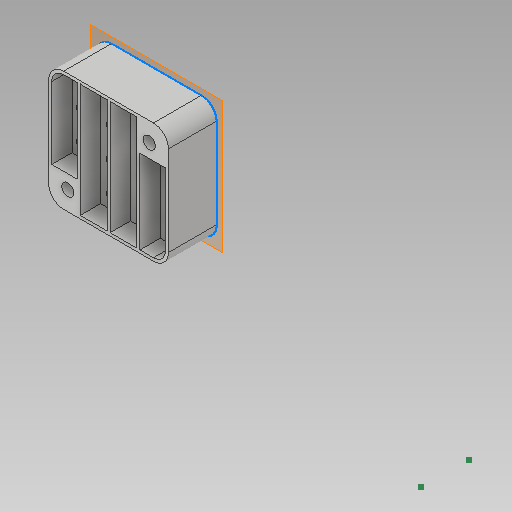
# Autodesk Inventor part: caster_wheel_1_inner
Saved by Autodesk Inventor 2019.3 (Build 233278000, 278)
## iProperties
Created: 2019-03-27
Part Number: caster_wheel_1_inner
Material: Generic
Document SubType Name: Modeling
Designer: Varga Daniel
Density: 1 g/cm^3
Appearance: Default
Author: Varga Daniel
Autodesk Inventor part; units mm, degrees
ref_plane "YZ Plane" through (0, 0, 0) normal (1, 0, 0) x (0, 1, 0)
ref_plane "XZ Plane" through (0, 0, 0) normal (0, 1, 0) x (-1, 0, 0)
ref_plane "Work Plane1" through (-90.2539, 56.452, 0) normal (0, 0, 1) x (1, 0, 0)
sketch "Sketch1" plane through (-90.2539, 56.452, 0) normal (0, 0, 1) x (1, 0, 0)
  arc A0 (0.6966, -35.7262) -> (5.6966, -30.7262) centre (0.6966, -30.7262) ccw
  line L0 (5.6966, -30.7262) -> (5.6966, -0.7262)
  arc A1 (5.6966, -0.7262) -> (0.6966, 4.2738) centre (0.6966, -0.7262) ccw
  line L1 (0.6966, 4.2738) -> (-29.3034, 4.2738)
  arc A2 (-29.3034, 4.2738) -> (-34.3034, -0.7262) centre (-29.3034, -0.7262) ccw
  line L2 (-34.3034, -0.7262) -> (-34.3034, -30.7262)
  arc A3 (-34.3034, -30.7262) -> (-29.3034, -35.7262) centre (-29.3034, -30.7262) ccw
  line L3 (-29.3034, -35.7262) -> (0.6966, -35.7262)
  line L4 (4.6966, -0.7262) -> (4.6966, -30.7262)
  arc A4 (0.6966, -34.7262) -> (4.6966, -30.7262) centre (0.6966, -30.7262) ccw
  line L5 (0.6966, -34.7262) -> (-3.8034, -34.7262)
  line L6 (-3.8034, -34.7262) -> (-3.8034, 3.2738)
  line L7 (-3.8034, 3.2738) -> (0.6966, 3.2738)
  arc A5 (4.6966, -0.7262) -> (0.6966, 3.2738) centre (0.6966, -0.7262) ccw
  line L8 (-4.8034, -34.7262) -> (-13.8034, -34.7262)
  line L9 (-13.8034, -34.7262) -> (-13.8034, 3.2738)
  line L10 (-13.8034, 3.2738) -> (-4.8034, 3.2738)
  line L11 (-4.8034, 3.2738) -> (-4.8034, -34.7262)
  line L12 (-14.8034, -34.7262) -> (-23.8034, -34.7262)
  line L13 (-23.8034, -34.7262) -> (-23.8034, 3.2738)
  line L14 (-23.8034, 3.2738) -> (-14.8034, 3.2738)
  line L15 (-14.8034, 3.2738) -> (-14.8034, -34.7262)
  line L16 (-33.3034, -30.7262) -> (-33.3034, -0.7262)
  arc A6 (-29.3034, 3.2738) -> (-33.3034, -0.7262) centre (-29.3034, -0.7262) ccw
  line L17 (-29.3034, 3.2738) -> (-24.8034, 3.2738)
  line L18 (-24.8034, 3.2738) -> (-24.8034, -34.7262)
  line L19 (-24.8034, -34.7262) -> (-29.3034, -34.7262)
  arc A7 (-33.3034, -30.7262) -> (-29.3034, -34.7262) centre (-29.3034, -30.7262) ccw
  line L20 (-28.8034, -7.2621) -> (-28.8034, -4.1903)
  arc A8 (-28.8034, -4.1903) -> (-25.8393, -1.2262) centre (-29.3034, -0.7262) ccw
  line L21 (-25.8393, -1.2262) -> (-24.8034, -1.2262)
  line L22 (-24.8034, -0.2262) -> (-24.8034, -1.2262)
  line L23 (-24.8034, -0.2262) -> (-25.8393, -0.2262)
  arc A9 (-25.8393, -0.2262) -> (-28.8034, 2.7379) centre (-29.3034, -0.7262) ccw
  line L24 (-28.8034, 2.7379) -> (-28.8034, 3.2738)
  line L25 (-29.3034, 3.2738) -> (-28.8034, 3.2738)
  arc A10 (-29.3034, 3.2738) -> (-29.8034, 3.2424) centre (-29.3034, -0.7262) ccw
  line L26 (-29.8034, 3.2424) -> (-29.8034, 2.7379)
  arc A11 (-29.8034, 2.7379) -> (-32.7675, -0.2262) centre (-29.3034, -0.7262) ccw
  line L27 (-32.7675, -0.2262) -> (-33.272, -0.2262)
  arc A12 (-33.272, -0.2262) -> (-33.3034, -0.7262) centre (-29.3034, -0.7262) ccw
  line L28 (-33.3034, -1.2262) -> (-33.3034, -0.7262)
  line L29 (-33.3034, -1.2262) -> (-32.7675, -1.2262)
  arc A13 (-32.7675, -1.2262) -> (-29.8034, -4.1903) centre (-29.3034, -0.7262) ccw
  line L30 (-29.8034, -4.1903) -> (-29.8034, -7.2621)
  arc A14 (-29.8034, -7.2621) -> (-32.7675, -10.2262) centre (-29.3034, -10.7262) ccw
  line L31 (-32.7675, -10.2262) -> (-33.3034, -10.2262)
  line L32 (-33.3034, -11.2262) -> (-33.3034, -10.2262)
  line L33 (-33.3034, -11.2262) -> (-32.7675, -11.2262)
  arc A15 (-32.7675, -11.2262) -> (-29.8034, -14.1903) centre (-29.3034, -10.7262) ccw
  line L34 (-29.8034, -14.1903) -> (-29.8034, -17.2621)
  arc A16 (-29.8034, -17.2621) -> (-32.7675, -20.2262) centre (-29.3034, -20.7262) ccw
  line L35 (-32.7675, -20.2262) -> (-33.3034, -20.2262)
  line L36 (-33.3034, -21.2262) -> (-33.3034, -20.2262)
  line L37 (-33.3034, -21.2262) -> (-32.7675, -21.2262)
  arc A17 (-32.7675, -21.2262) -> (-29.8034, -24.1903) centre (-29.3034, -20.7262) ccw
  line L38 (-29.8034, -24.1903) -> (-29.8034, -27.2621)
  arc A18 (-29.8034, -27.2621) -> (-32.7675, -30.2262) centre (-29.3034, -30.7262) ccw
  line L39 (-32.7675, -30.2262) -> (-33.3034, -30.2262)
  line L40 (-33.3034, -30.7262) -> (-33.3034, -30.2262)
  arc A19 (-33.3034, -30.7262) -> (-33.272, -31.2262) centre (-29.3034, -30.7262) ccw
  line L41 (-33.272, -31.2262) -> (-32.7675, -31.2262)
  arc A20 (-32.7675, -31.2262) -> (-29.8034, -34.1903) centre (-29.3034, -30.7262) ccw
  line L42 (-29.8034, -34.1903) -> (-29.8034, -34.6949)
  arc A21 (-29.8034, -34.6949) -> (-29.3034, -34.7262) centre (-29.3034, -30.7262) ccw
  line L43 (-28.8034, -34.7262) -> (-29.3034, -34.7262)
  line L44 (-28.8034, -34.7262) -> (-28.8034, -34.1903)
  arc A22 (-28.8034, -34.1903) -> (-25.8393, -31.2262) centre (-29.3034, -30.7262) ccw
  line L45 (-25.8393, -31.2262) -> (-24.8034, -31.2262)
  line L46 (-24.8034, -30.2262) -> (-24.8034, -31.2262)
  line L47 (-24.8034, -30.2262) -> (-25.8393, -30.2262)
  arc A23 (-25.8393, -30.2262) -> (-28.8034, -27.2621) centre (-29.3034, -30.7262) ccw
  line L48 (-28.8034, -27.2621) -> (-28.8034, -24.1903)
  arc A24 (-28.8034, -24.1903) -> (-25.8393, -21.2262) centre (-29.3034, -20.7262) ccw
  line L49 (-25.8393, -21.2262) -> (-24.8034, -21.2262)
  line L50 (-24.8034, -20.2262) -> (-24.8034, -21.2262)
  line L51 (-24.8034, -20.2262) -> (-25.8393, -20.2262)
  arc A25 (-25.8393, -20.2262) -> (-28.8034, -17.2621) centre (-29.3034, -20.7262) ccw
  line L52 (-28.8034, -17.2621) -> (-28.8034, -14.1903)
  arc A26 (-28.8034, -14.1903) -> (-25.8393, -11.2262) centre (-29.3034, -10.7262) ccw
  line L53 (-25.8393, -11.2262) -> (-24.8034, -11.2262)
  line L54 (-24.8034, -10.2262) -> (-24.8034, -11.2262)
  line L55 (-24.8034, -10.2262) -> (-25.8393, -10.2262)
  arc A27 (-25.8393, -10.2262) -> (-28.8034, -7.2621) centre (-29.3034, -10.7262) ccw
  circle A28 centre (-29.3034, -10.7262) radius 2.5
  circle A29 centre (-29.3034, -20.7262) radius 2.5
  circle A30 centre (-29.3034, -30.7262) radius 2.5
  circle A31 centre (-29.3034, -0.7262) radius 2.5
  line L56 (-22.7675, -0.2262) -> (-23.8034, -0.2262)
  line L57 (-23.8034, -1.2262) -> (-23.8034, -0.2262)
  line L58 (-23.8034, -1.2262) -> (-22.7675, -1.2262)
  arc A32 (-22.7675, -1.2262) -> (-19.8034, -4.1903) centre (-19.3034, -0.7262) ccw
  line L59 (-19.8034, -4.1903) -> (-19.8034, -7.2621)
  arc A33 (-19.8034, -7.2621) -> (-22.7675, -10.2262) centre (-19.3034, -10.7262) ccw
  line L60 (-22.7675, -10.2262) -> (-23.8034, -10.2262)
  line L61 (-23.8034, -11.2262) -> (-23.8034, -10.2262)
  line L62 (-23.8034, -11.2262) -> (-22.7675, -11.2262)
  arc A34 (-22.7675, -11.2262) -> (-19.8034, -14.1903) centre (-19.3034, -10.7262) ccw
  line L63 (-19.8034, -14.1903) -> (-19.8034, -17.2621)
  arc A35 (-19.8034, -17.2621) -> (-22.7675, -20.2262) centre (-19.3034, -20.7262) ccw
  line L64 (-22.7675, -20.2262) -> (-23.8034, -20.2262)
  line L65 (-23.8034, -21.2262) -> (-23.8034, -20.2262)
  line L66 (-23.8034, -21.2262) -> (-22.7675, -21.2262)
  arc A36 (-22.7675, -21.2262) -> (-19.8034, -24.1903) centre (-19.3034, -20.7262) ccw
  line L67 (-19.8034, -24.1903) -> (-19.8034, -27.2621)
  arc A37 (-19.8034, -27.2621) -> (-22.7675, -30.2262) centre (-19.3034, -30.7262) ccw
  line L68 (-22.7675, -30.2262) -> (-23.8034, -30.2262)
  line L69 (-23.8034, -31.2262) -> (-23.8034, -30.2262)
  line L70 (-23.8034, -31.2262) -> (-22.7675, -31.2262)
  arc A38 (-22.7675, -31.2262) -> (-19.8034, -34.1903) centre (-19.3034, -30.7262) ccw
  line L71 (-19.8034, -34.1903) -> (-19.8034, -34.7262)
  line L72 (-18.8034, -34.7262) -> (-19.8034, -34.7262)
  line L73 (-18.8034, -34.7262) -> (-18.8034, -34.1903)
  arc A39 (-18.8034, -34.1903) -> (-15.8393, -31.2262) centre (-19.3034, -30.7262) ccw
  line L74 (-15.8393, -31.2262) -> (-14.8034, -31.2262)
  line L75 (-14.8034, -30.2262) -> (-14.8034, -31.2262)
  line L76 (-14.8034, -30.2262) -> (-15.8393, -30.2262)
  arc A40 (-15.8393, -30.2262) -> (-18.8034, -27.2621) centre (-19.3034, -30.7262) ccw
  line L77 (-18.8034, -27.2621) -> (-18.8034, -24.1903)
  arc A41 (-18.8034, -24.1903) -> (-15.8393, -21.2262) centre (-19.3034, -20.7262) ccw
  line L78 (-15.8393, -21.2262) -> (-14.8034, -21.2262)
  line L79 (-14.8034, -20.2262) -> (-14.8034, -21.2262)
  line L80 (-14.8034, -20.2262) -> (-15.8393, -20.2262)
  arc A42 (-15.8393, -20.2262) -> (-18.8034, -17.2621) centre (-19.3034, -20.7262) ccw
  line L81 (-18.8034, -17.2621) -> (-18.8034, -14.1903)
  arc A43 (-18.8034, -14.1903) -> (-15.8393, -11.2262) centre (-19.3034, -10.7262) ccw
  line L82 (-15.8393, -11.2262) -> (-14.8034, -11.2262)
  line L83 (-14.8034, -10.2262) -> (-14.8034, -11.2262)
  line L84 (-14.8034, -10.2262) -> (-15.8393, -10.2262)
  arc A44 (-15.8393, -10.2262) -> (-18.8034, -7.2621) centre (-19.3034, -10.7262) ccw
  line L85 (-18.8034, -7.2621) -> (-18.8034, -4.1903)
  arc A45 (-18.8034, -4.1903) -> (-15.8393, -1.2262) centre (-19.3034, -0.7262) ccw
  line L86 (-15.8393, -1.2262) -> (-14.8034, -1.2262)
  line L87 (-14.8034, -0.2262) -> (-14.8034, -1.2262)
  line L88 (-14.8034, -0.2262) -> (-15.8393, -0.2262)
  arc A46 (-15.8393, -0.2262) -> (-18.8034, 2.7379) centre (-19.3034, -0.7262) ccw
  line L89 (-18.8034, 2.7379) -> (-18.8034, 3.2738)
  line L90 (-19.8034, 3.2738) -> (-18.8034, 3.2738)
  line L91 (-19.8034, 3.2738) -> (-19.8034, 2.7379)
  arc A47 (-19.8034, 2.7379) -> (-22.7675, -0.2262) centre (-19.3034, -0.7262) ccw
  circle A48 centre (-19.3034, -10.7262) radius 2.5
  circle A49 centre (-19.3034, -20.7262) radius 2.5
  circle A50 centre (-19.3034, -30.7262) radius 2.5
  circle A51 centre (-19.3034, -0.7262) radius 2.5
  line L92 (-12.7675, -0.2262) -> (-13.8034, -0.2262)
  line L93 (-13.8034, -1.2262) -> (-13.8034, -0.2262)
  line L94 (-13.8034, -1.2262) -> (-12.7675, -1.2262)
  arc A52 (-12.7675, -1.2262) -> (-9.8034, -4.1903) centre (-9.3034, -0.7262) ccw
  line L95 (-9.8034, -4.1903) -> (-9.8034, -7.2621)
  arc A53 (-9.8034, -7.2621) -> (-12.7675, -10.2262) centre (-9.3034, -10.7262) ccw
  line L96 (-12.7675, -10.2262) -> (-13.8034, -10.2262)
  line L97 (-13.8034, -11.2262) -> (-13.8034, -10.2262)
  line L98 (-13.8034, -11.2262) -> (-12.7675, -11.2262)
  arc A54 (-12.7675, -11.2262) -> (-9.8034, -14.1903) centre (-9.3034, -10.7262) ccw
  line L99 (-9.8034, -14.1903) -> (-9.8034, -17.2621)
  arc A55 (-9.8034, -17.2621) -> (-12.7675, -20.2262) centre (-9.3034, -20.7262) ccw
  line L100 (-12.7675, -20.2262) -> (-13.8034, -20.2262)
  line L101 (-13.8034, -21.2262) -> (-13.8034, -20.2262)
  line L102 (-13.8034, -21.2262) -> (-12.7675, -21.2262)
  arc A56 (-12.7675, -21.2262) -> (-9.8034, -24.1903) centre (-9.3034, -20.7262) ccw
  line L103 (-9.8034, -24.1903) -> (-9.8034, -27.2621)
  arc A57 (-9.8034, -27.2621) -> (-12.7675, -30.2262) centre (-9.3034, -30.7262) ccw
  line L104 (-12.7675, -30.2262) -> (-13.8034, -30.2262)
  line L105 (-13.8034, -31.2262) -> (-13.8034, -30.2262)
  line L106 (-13.8034, -31.2262) -> (-12.7675, -31.2262)
  arc A58 (-12.7675, -31.2262) -> (-9.8034, -34.1903) centre (-9.3034, -30.7262) ccw
  line L107 (-9.8034, -34.1903) -> (-9.8034, -34.7262)
  line L108 (-8.8034, -34.7262) -> (-9.8034, -34.7262)
  line L109 (-8.8034, -34.7262) -> (-8.8034, -34.1903)
  arc A59 (-8.8034, -34.1903) -> (-5.8393, -31.2262) centre (-9.3034, -30.7262) ccw
  line L110 (-5.8393, -31.2262) -> (-4.8034, -31.2262)
  line L111 (-4.8034, -30.2262) -> (-4.8034, -31.2262)
  line L112 (-4.8034, -30.2262) -> (-5.8393, -30.2262)
  arc A60 (-5.8393, -30.2262) -> (-8.8034, -27.2621) centre (-9.3034, -30.7262) ccw
  line L113 (-8.8034, -27.2621) -> (-8.8034, -24.1903)
  arc A61 (-8.8034, -24.1903) -> (-5.8393, -21.2262) centre (-9.3034, -20.7262) ccw
  line L114 (-5.8393, -21.2262) -> (-4.8034, -21.2262)
  line L115 (-4.8034, -20.2262) -> (-4.8034, -21.2262)
  line L116 (-4.8034, -20.2262) -> (-5.8393, -20.2262)
  arc A62 (-5.8393, -20.2262) -> (-8.8034, -17.2621) centre (-9.3034, -20.7262) ccw
  line L117 (-8.8034, -17.2621) -> (-8.8034, -14.1903)
  arc A63 (-8.8034, -14.1903) -> (-5.8393, -11.2262) centre (-9.3034, -10.7262) ccw
  line L118 (-5.8393, -11.2262) -> (-4.8034, -11.2262)
  line L119 (-4.8034, -10.2262) -> (-4.8034, -11.2262)
  line L120 (-4.8034, -10.2262) -> (-5.8393, -10.2262)
  arc A64 (-5.8393, -10.2262) -> (-8.8034, -7.2621) centre (-9.3034, -10.7262) ccw
  line L121 (-8.8034, -7.2621) -> (-8.8034, -4.1903)
  arc A65 (-8.8034, -4.1903) -> (-5.8393, -1.2262) centre (-9.3034, -0.7262) ccw
  line L122 (-5.8393, -1.2262) -> (-4.8034, -1.2262)
  line L123 (-4.8034, -0.2262) -> (-4.8034, -1.2262)
  line L124 (-4.8034, -0.2262) -> (-5.8393, -0.2262)
  arc A66 (-5.8393, -0.2262) -> (-8.8034, 2.7379) centre (-9.3034, -0.7262) ccw
  line L125 (-8.8034, 2.7379) -> (-8.8034, 3.2738)
  line L126 (-9.8034, 3.2738) -> (-8.8034, 3.2738)
  line L127 (-9.8034, 3.2738) -> (-9.8034, 2.7379)
  arc A67 (-9.8034, 2.7379) -> (-12.7675, -0.2262) centre (-9.3034, -0.7262) ccw
  circle A68 centre (-9.3034, -10.7262) radius 2.5
  circle A69 centre (-9.3034, -20.7262) radius 2.5
  circle A70 centre (-9.3034, -30.7262) radius 2.5
  circle A71 centre (-9.3034, -0.7262) radius 2.5
  line L128 (0.1966, -4.1903) -> (0.1966, -7.2621)
  arc A72 (0.1966, -7.2621) -> (-2.7675, -10.2262) centre (0.6966, -10.7262) ccw
  line L129 (-2.7675, -10.2262) -> (-3.8034, -10.2262)
  line L130 (-3.8034, -11.2262) -> (-3.8034, -10.2262)
  line L131 (-3.8034, -11.2262) -> (-2.7675, -11.2262)
  arc A73 (-2.7675, -11.2262) -> (0.1966, -14.1903) centre (0.6966, -10.7262) ccw
  line L132 (0.1966, -14.1903) -> (0.1966, -17.2621)
  arc A74 (0.1966, -17.2621) -> (-2.7675, -20.2262) centre (0.6966, -20.7262) ccw
  line L133 (-2.7675, -20.2262) -> (-3.8034, -20.2262)
  line L134 (-3.8034, -21.2262) -> (-3.8034, -20.2262)
  line L135 (-3.8034, -21.2262) -> (-2.7675, -21.2262)
  arc A75 (-2.7675, -21.2262) -> (0.1966, -24.1903) centre (0.6966, -20.7262) ccw
  line L136 (0.1966, -24.1903) -> (0.1966, -27.2621)
  arc A76 (0.1966, -27.2621) -> (-2.7675, -30.2262) centre (0.6966, -30.7262) ccw
  line L137 (-2.7675, -30.2262) -> (-3.8034, -30.2262)
  line L138 (-3.8034, -31.2262) -> (-3.8034, -30.2262)
  line L139 (-3.8034, -31.2262) -> (-2.7675, -31.2262)
  arc A77 (-2.7675, -31.2262) -> (0.1966, -34.1903) centre (0.6966, -30.7262) ccw
  line L140 (0.1966, -34.1903) -> (0.1966, -34.7262)
  line L141 (0.6966, -34.7262) -> (0.1966, -34.7262)
  arc A78 (0.6966, -34.7262) -> (1.1966, -34.6949) centre (0.6966, -30.7262) ccw
  line L142 (1.1966, -34.6949) -> (1.1966, -34.1903)
  arc A79 (1.1966, -34.1903) -> (4.1607, -31.2262) centre (0.6966, -30.7262) ccw
  line L143 (4.1607, -31.2262) -> (4.6652, -31.2262)
  arc A80 (4.6652, -31.2262) -> (4.6966, -30.7262) centre (0.6966, -30.7262) ccw
  line L144 (4.6966, -30.2262) -> (4.6966, -30.7262)
  line L145 (4.6966, -30.2262) -> (4.1607, -30.2262)
  arc A81 (4.1607, -30.2262) -> (1.1966, -27.2621) centre (0.6966, -30.7262) ccw
  line L146 (1.1966, -27.2621) -> (1.1966, -24.1903)
  arc A82 (1.1966, -24.1903) -> (4.1607, -21.2262) centre (0.6966, -20.7262) ccw
  line L147 (4.1607, -21.2262) -> (4.6966, -21.2262)
  line L148 (4.6966, -20.2262) -> (4.6966, -21.2262)
  line L149 (4.6966, -20.2262) -> (4.1607, -20.2262)
  arc A83 (4.1607, -20.2262) -> (1.1966, -17.2621) centre (0.6966, -20.7262) ccw
  line L150 (1.1966, -17.2621) -> (1.1966, -14.1903)
  arc A84 (1.1966, -14.1903) -> (4.1607, -11.2262) centre (0.6966, -10.7262) ccw
  line L151 (4.1607, -11.2262) -> (4.6966, -11.2262)
  line L152 (4.6966, -10.2262) -> (4.6966, -11.2262)
  line L153 (4.6966, -10.2262) -> (4.1607, -10.2262)
  arc A85 (4.1607, -10.2262) -> (1.1966, -7.2621) centre (0.6966, -10.7262) ccw
  line L154 (1.1966, -7.2621) -> (1.1966, -4.1903)
  arc A86 (1.1966, -4.1903) -> (4.1607, -1.2262) centre (0.6966, -0.7262) ccw
  line L155 (4.1607, -1.2262) -> (4.6966, -1.2262)
  line L156 (4.6966, -0.7262) -> (4.6966, -1.2262)
  arc A87 (4.6966, -0.7262) -> (4.6652, -0.2262) centre (0.6966, -0.7262) ccw
  line L157 (4.6652, -0.2262) -> (4.1607, -0.2262)
  arc A88 (4.1607, -0.2262) -> (1.1966, 2.7379) centre (0.6966, -0.7262) ccw
  line L158 (1.1966, 2.7379) -> (1.1966, 3.2424)
  arc A89 (1.1966, 3.2424) -> (0.6966, 3.2738) centre (0.6966, -0.7262) ccw
  line L159 (0.1966, 3.2738) -> (0.6966, 3.2738)
  line L160 (0.1966, 3.2738) -> (0.1966, 2.7379)
  arc A90 (0.1966, 2.7379) -> (-2.7675, -0.2262) centre (0.6966, -0.7262) ccw
  line L161 (-2.7675, -0.2262) -> (-3.8034, -0.2262)
  line L162 (-3.8034, -1.2262) -> (-3.8034, -0.2262)
  line L163 (-3.8034, -1.2262) -> (-2.7675, -1.2262)
  arc A91 (-2.7675, -1.2262) -> (0.1966, -4.1903) centre (0.6966, -0.7262) ccw
  circle A92 centre (0.6966, -10.7262) radius 2.5
  circle A93 centre (0.6966, -20.7262) radius 2.5
  circle A94 centre (0.6966, -30.7262) radius 2.5
  circle A95 centre (0.6966, -0.7262) radius 2.5
  point P0 (90.2539, -56.452)
  constraints: 316 end point, 160 point on circle, 96 centre point, 18 other
extrude "Extrusion2" add sketch "Sketch1" along normal blind 16 contours L4 L155 A86 L154 A85 L153 L151 A84 L150 A83 L149 L147 A82 L146 A81 L145 A4 L143 A79 L142 L5 L140 A77 L139 L6 L137 A76 L136 A75 L135 L133 A74 L132 A73 L131 L129 A72 L128 A91 L163 L161 A90 L160 L7 A5 L158 A88 L157 | L4 L153 A85 L154 A86 L155 | L157 A88 L158 A5 | L4 L149 A83 L150 A84 L151 | L160 A90 L161 L6 L7 | L4 L145 A81 L146 A82 L147 | L163 A91 L128 A72 L129 L6 | A4 L142 A79 L143 | L131 A73 L132 A74 L133 L6 | L5 L6 L139 A77 L140 | L135 A75 L136 A76 L137 L6 | L8 L109 A59 L110 L11 | L8 L107 A58 L106 L9 L104 A57 L103 A56 L102 L100 A55 L99 A54 L98 L96 A53 L95 A52 L94 L92 A67 L127 L10 L125 A66 L124 L11 L122 A65 L121 A64 L120 L118 A63 L117 A62 L116 L114 A61 L113 A60 L112 L110 A59 L109 | L8 L9 L106 A58 L107 | L112 A60 L113 A61 L114 L11 | L116 A62 L117 A63 L118 L11 | L9 L102 A56 L103 A57 L104 | L120 A64 L121 A65 L122 L11 | L9 L98 A54 L99 A55 L100 | L124 A66 L125 L10 L11 | L9 L94 A52 L95 A53 L96 | L9 L10 L127 A67 L92 | L12 L73 A39 L74 L15 | L12 L71 A38 L70 L13 L68 A37 L67 A36 L66 L64 A35 L63 A34 L62 L60 A33 L59 A32 L58 L56 A47 L91 L14 L89 A46 L88 L15 L86 A45 L85 A44 L84 L82 A43 L81 A42 L80 L78 A41 L77 A40 L76 L74 A39 L73 | L12 L13 L70 A38 L71 | L76 A40 L77 A41 L78 L15 | L80 A42 L81 A43 L82 L15 | L13 L66 A36 L67 A37 L68 | L84 A44 L85 A45 L86 L15 | L13 L62 A34 L63 A35 L64 | L88 A46 L89 L14 L15 | L13 L58 A32 L59 A33 L60 | L13 L14 L91 A47 L56 | L16 L39 A18 L38 A17 L37 L35 A16 L34 A15 L33 L31 A14 L30 A13 L29 A6 L27 A11 L26 L17 L24 A9 L23 L18 L21 A8 L20 A27 L55 L53 A26 L52 A25 L51 L49 A24 L48 A23 L47 L45 A22 L44 L19 A7 L42 A20 L41 | L16 L37 A17 L38 A18 L39 | L41 A20 L42 A7 | L16 L33 A15 L34 A16 L35 | L44 A22 L45 L18 L19 | L16 L29 A13 L30 A14 L31 | L47 A23 L48 A24 L49 L18 | A6 L26 A11 L27 | L51 A25 L52 A26 L53 L18 | L17 L18 L23 A9 L24 | L55 A27 L20 A8 L21 L18 | A28 | A29 | A30 | A31 | A48 | A49 | A50 | A51 | A68 | A69 | A70 | A71 | A92 | A93 | A94 | A95
extrude "Extrusion3" add sketch "Sketch1" along normal blind 16 contours L3 A3 L2 A2 L1 A1 L0 A0
extrude "Extrusion4" cut sketch "Sketch1" along normal blind 0.8 contours L4 L155 A86 L154 A85 L153 L151 A84 L150 A83 L149 L147 A82 L146 A81 L145 A4 L143 A79 L142 L5 L140 A77 L139 L6 L137 A76 L136 A75 L135 L133 A74 L132 A73 L131 L129 A72 L128 A91 L163 L161 A90 L160 L7 A5 L158 A88 L157 | L4 L153 A85 L154 A86 L155 | L157 A88 L158 A5 | L4 L149 A83 L150 A84 L151 | L160 A90 L161 L6 L7 | L4 L145 A81 L146 A82 L147 | L163 A91 L128 A72 L129 L6 | A4 L142 A79 L143 | L131 A73 L132 A74 L133 L6 | L5 L6 L139 A77 L140 | L135 A75 L136 A76 L137 L6 | L8 L109 A59 L110 L11 | L8 L107 A58 L106 L9 L104 A57 L103 A56 L102 L100 A55 L99 A54 L98 L96 A53 L95 A52 L94 L92 A67 L127 L10 L125 A66 L124 L11 L122 A65 L121 A64 L120 L118 A63 L117 A62 L116 L114 A61 L113 A60 L112 L110 A59 L109 | L8 L9 L106 A58 L107 | L112 A60 L113 A61 L114 L11 | L116 A62 L117 A63 L118 L11 | L9 L102 A56 L103 A57 L104 | L120 A64 L121 A65 L122 L11 | L9 L98 A54 L99 A55 L100 | L124 A66 L125 L10 L11 | L9 L94 A52 L95 A53 L96 | L9 L10 L127 A67 L92 | L12 L73 A39 L74 L15 | L12 L71 A38 L70 L13 L68 A37 L67 A36 L66 L64 A35 L63 A34 L62 L60 A33 L59 A32 L58 L56 A47 L91 L14 L89 A46 L88 L15 L86 A45 L85 A44 L84 L82 A43 L81 A42 L80 L78 A41 L77 A40 L76 L74 A39 L73 | L12 L13 L70 A38 L71 | L76 A40 L77 A41 L78 L15 | L80 A42 L81 A43 L82 L15 | L13 L66 A36 L67 A37 L68 | L84 A44 L85 A45 L86 L15 | L13 L62 A34 L63 A35 L64 | L88 A46 L89 L14 L15 | L13 L58 A32 L59 A33 L60 | L13 L14 L91 A47 L56 | L16 L39 A18 L38 A17 L37 L35 A16 L34 A15 L33 L31 A14 L30 A13 L29 A6 L27 A11 L26 L17 L24 A9 L23 L18 L21 A8 L20 A27 L55 L53 A26 L52 A25 L51 L49 A24 L48 A23 L47 L45 A22 L44 L19 A7 L42 A20 L41 | L16 L37 A17 L38 A18 L39 | L41 A20 L42 A7 | L16 L33 A15 L34 A16 L35 | L44 A22 L45 L18 L19 | L16 L29 A13 L30 A14 L31 | L47 A23 L48 A24 L49 L18 | A6 L26 A11 L27 | L51 A25 L52 A26 L53 L18 | L17 L18 L23 A9 L24 | L55 A27 L20 A8 L21 L18 | A28 | A29 | A30 | A31 | A48 | A49 | A50 | A51 | A68 | A69 | A70 | A71 | A92 | A93 | A94 | A95
extrude "Extrusion5" cut sketch "Sketch1" along normal blind 9.2 contours A28 | A29 | A31 | A48 | A49 | A50 | A51 | A68 | A69 | A70 | A71 | A92 | A93 | A94
sketch "Sketch2" plane through (-90.2539, 56.452, 16) normal (0, 0, 1) x (1, 0, 0)
  point P0 (90.2539, -56.452)
sketch "Sketch3" plane through (-90.2539, 56.452, 16) normal (0, 0, 1) x (1, 0, 0)
  arc A0 (-29.3034, 4.2738) -> (-34.3034, -0.7262) centre (-29.3034, -0.7262) ccw
  line L0 (-29.3034, 4.2738) -> (0.6966, 4.2738)
  arc A1 (5.6966, -0.7262) -> (0.6966, 4.2738) centre (0.6966, -0.7262) ccw
  line L1 (5.6966, -0.7262) -> (5.6966, -30.7262)
  arc A2 (0.6966, -35.7262) -> (5.6966, -30.7262) centre (0.6966, -30.7262) ccw
  line L2 (0.6966, -35.7262) -> (-29.3034, -35.7262)
  arc A3 (-34.3034, -30.7262) -> (-29.3034, -35.7262) centre (-29.3034, -30.7262) ccw
  line L3 (-34.3034, -30.7262) -> (-34.3034, -0.7262)
  line L4 (4.6966, -30.7262) -> (4.6966, -0.7262)
  arc A4 (4.6966, -0.7262) -> (0.6966, 3.2738) centre (0.6966, -0.7262) ccw
  line L5 (0.6966, 3.2738) -> (-3.8034, 3.2738)
  line L6 (-3.8034, 3.2738) -> (-3.8034, -34.7262)
  line L7 (-3.8034, -34.7262) -> (0.6966, -34.7262)
  arc A5 (0.6966, -34.7262) -> (4.6966, -30.7262) centre (0.6966, -30.7262) ccw
  line L8 (-13.8034, -34.7262) -> (-4.8034, -34.7262)
  line L9 (-4.8034, -34.7262) -> (-4.8034, 3.2738)
  line L10 (-4.8034, 3.2738) -> (-13.8034, 3.2738)
  line L11 (-13.8034, 3.2738) -> (-13.8034, -34.7262)
  line L12 (-23.8034, -34.7262) -> (-14.8034, -34.7262)
  line L13 (-14.8034, -34.7262) -> (-14.8034, 3.2738)
  line L14 (-14.8034, 3.2738) -> (-23.8034, 3.2738)
  line L15 (-23.8034, 3.2738) -> (-23.8034, -34.7262)
  line L16 (-33.3034, -0.7262) -> (-33.3034, -30.7262)
  arc A6 (-33.3034, -30.7262) -> (-29.3034, -34.7262) centre (-29.3034, -30.7262) ccw
  line L17 (-29.3034, -34.7262) -> (-24.8034, -34.7262)
  line L18 (-24.8034, -34.7262) -> (-24.8034, 3.2738)
  line L19 (-24.8034, 3.2738) -> (-29.3034, 3.2738)
  arc A7 (-29.3034, 3.2738) -> (-33.3034, -0.7262) centre (-29.3034, -0.7262) ccw
  line L20 (-28.8034, -4.1903) -> (-28.8034, -7.2621)
  arc A8 (-25.8393, -10.2262) -> (-28.8034, -7.2621) centre (-29.3034, -10.7262) ccw
  line L21 (-25.8393, -10.2262) -> (-24.8034, -10.2262)
  line L22 (-24.8034, -11.2262) -> (-24.8034, -10.2262)
  line L23 (-24.8034, -11.2262) -> (-25.8393, -11.2262)
  arc A9 (-28.8034, -14.1903) -> (-25.8393, -11.2262) centre (-29.3034, -10.7262) ccw
  line L24 (-28.8034, -14.1903) -> (-28.8034, -17.2621)
  arc A10 (-25.8393, -20.2262) -> (-28.8034, -17.2621) centre (-29.3034, -20.7262) ccw
  line L25 (-25.8393, -20.2262) -> (-24.8034, -20.2262)
  line L26 (-24.8034, -21.2262) -> (-24.8034, -20.2262)
  line L27 (-24.8034, -21.2262) -> (-25.8393, -21.2262)
  arc A11 (-28.8034, -24.1903) -> (-25.8393, -21.2262) centre (-29.3034, -20.7262) ccw
  line L28 (-28.8034, -24.1903) -> (-28.8034, -27.2621)
  arc A12 (-25.8393, -30.2262) -> (-28.8034, -27.2621) centre (-29.3034, -30.7262) ccw
  line L29 (-25.8393, -30.2262) -> (-24.8034, -30.2262)
  line L30 (-24.8034, -31.2262) -> (-24.8034, -30.2262)
  line L31 (-24.8034, -31.2262) -> (-25.8393, -31.2262)
  arc A13 (-28.8034, -34.1903) -> (-25.8393, -31.2262) centre (-29.3034, -30.7262) ccw
  line L32 (-28.8034, -34.1903) -> (-28.8034, -34.7262)
  line L33 (-29.3034, -34.7262) -> (-28.8034, -34.7262)
  arc A14 (-29.8034, -34.6949) -> (-29.3034, -34.7262) centre (-29.3034, -30.7262) ccw
  line L34 (-29.8034, -34.6949) -> (-29.8034, -34.1903)
  arc A15 (-32.7675, -31.2262) -> (-29.8034, -34.1903) centre (-29.3034, -30.7262) ccw
  line L35 (-32.7675, -31.2262) -> (-33.272, -31.2262)
  arc A16 (-33.3034, -30.7262) -> (-33.272, -31.2262) centre (-29.3034, -30.7262) ccw
  line L36 (-33.3034, -30.2262) -> (-33.3034, -30.7262)
  line L37 (-33.3034, -30.2262) -> (-32.7675, -30.2262)
  arc A17 (-29.8034, -27.2621) -> (-32.7675, -30.2262) centre (-29.3034, -30.7262) ccw
  line L38 (-29.8034, -27.2621) -> (-29.8034, -24.1903)
  arc A18 (-32.7675, -21.2262) -> (-29.8034, -24.1903) centre (-29.3034, -20.7262) ccw
  line L39 (-32.7675, -21.2262) -> (-33.3034, -21.2262)
  line L40 (-33.3034, -20.2262) -> (-33.3034, -21.2262)
  line L41 (-33.3034, -20.2262) -> (-32.7675, -20.2262)
  arc A19 (-29.8034, -17.2621) -> (-32.7675, -20.2262) centre (-29.3034, -20.7262) ccw
  line L42 (-29.8034, -17.2621) -> (-29.8034, -14.1903)
  arc A20 (-32.7675, -11.2262) -> (-29.8034, -14.1903) centre (-29.3034, -10.7262) ccw
  line L43 (-32.7675, -11.2262) -> (-33.3034, -11.2262)
  line L44 (-33.3034, -10.2262) -> (-33.3034, -11.2262)
  line L45 (-33.3034, -10.2262) -> (-32.7675, -10.2262)
  arc A21 (-29.8034, -7.2621) -> (-32.7675, -10.2262) centre (-29.3034, -10.7262) ccw
  line L46 (-29.8034, -7.2621) -> (-29.8034, -4.1903)
  arc A22 (-32.7675, -1.2262) -> (-29.8034, -4.1903) centre (-29.3034, -0.7262) ccw
  line L47 (-32.7675, -1.2262) -> (-33.3034, -1.2262)
  line L48 (-33.3034, -0.7262) -> (-33.3034, -1.2262)
  arc A23 (-33.272, -0.2262) -> (-33.3034, -0.7262) centre (-29.3034, -0.7262) ccw
  line L49 (-33.272, -0.2262) -> (-32.7675, -0.2262)
  arc A24 (-29.8034, 2.7379) -> (-32.7675, -0.2262) centre (-29.3034, -0.7262) ccw
  line L50 (-29.8034, 2.7379) -> (-29.8034, 3.2424)
  arc A25 (-29.3034, 3.2738) -> (-29.8034, 3.2424) centre (-29.3034, -0.7262) ccw
  line L51 (-28.8034, 3.2738) -> (-29.3034, 3.2738)
  line L52 (-28.8034, 3.2738) -> (-28.8034, 2.7379)
  arc A26 (-25.8393, -0.2262) -> (-28.8034, 2.7379) centre (-29.3034, -0.7262) ccw
  line L53 (-25.8393, -0.2262) -> (-24.8034, -0.2262)
  line L54 (-24.8034, -1.2262) -> (-24.8034, -0.2262)
  line L55 (-24.8034, -1.2262) -> (-25.8393, -1.2262)
  arc A27 (-28.8034, -4.1903) -> (-25.8393, -1.2262) centre (-29.3034, -0.7262) ccw
  circle A28 centre (-29.3034, -10.7262) radius 2.5
  circle A29 centre (-29.3034, -20.7262) radius 2.5
  circle A30 centre (-29.3034, -30.7262) radius 2.5
  circle A31 centre (-29.3034, -0.7262) radius 2.5
  line L56 (-23.8034, -0.2262) -> (-22.7675, -0.2262)
  arc A32 (-19.8034, 2.7379) -> (-22.7675, -0.2262) centre (-19.3034, -0.7262) ccw
  line L57 (-19.8034, 2.7379) -> (-19.8034, 3.2738)
  line L58 (-18.8034, 3.2738) -> (-19.8034, 3.2738)
  line L59 (-18.8034, 3.2738) -> (-18.8034, 2.7379)
  arc A33 (-15.8393, -0.2262) -> (-18.8034, 2.7379) centre (-19.3034, -0.7262) ccw
  line L60 (-15.8393, -0.2262) -> (-14.8034, -0.2262)
  line L61 (-14.8034, -1.2262) -> (-14.8034, -0.2262)
  line L62 (-14.8034, -1.2262) -> (-15.8393, -1.2262)
  arc A34 (-18.8034, -4.1903) -> (-15.8393, -1.2262) centre (-19.3034, -0.7262) ccw
  line L63 (-18.8034, -4.1903) -> (-18.8034, -7.2621)
  arc A35 (-15.8393, -10.2262) -> (-18.8034, -7.2621) centre (-19.3034, -10.7262) ccw
  line L64 (-15.8393, -10.2262) -> (-14.8034, -10.2262)
  line L65 (-14.8034, -11.2262) -> (-14.8034, -10.2262)
  line L66 (-14.8034, -11.2262) -> (-15.8393, -11.2262)
  arc A36 (-18.8034, -14.1903) -> (-15.8393, -11.2262) centre (-19.3034, -10.7262) ccw
  line L67 (-18.8034, -14.1903) -> (-18.8034, -17.2621)
  arc A37 (-15.8393, -20.2262) -> (-18.8034, -17.2621) centre (-19.3034, -20.7262) ccw
  line L68 (-15.8393, -20.2262) -> (-14.8034, -20.2262)
  line L69 (-14.8034, -21.2262) -> (-14.8034, -20.2262)
  line L70 (-14.8034, -21.2262) -> (-15.8393, -21.2262)
  arc A38 (-18.8034, -24.1903) -> (-15.8393, -21.2262) centre (-19.3034, -20.7262) ccw
  line L71 (-18.8034, -24.1903) -> (-18.8034, -27.2621)
  arc A39 (-15.8393, -30.2262) -> (-18.8034, -27.2621) centre (-19.3034, -30.7262) ccw
  line L72 (-15.8393, -30.2262) -> (-14.8034, -30.2262)
  line L73 (-14.8034, -31.2262) -> (-14.8034, -30.2262)
  line L74 (-14.8034, -31.2262) -> (-15.8393, -31.2262)
  arc A40 (-18.8034, -34.1903) -> (-15.8393, -31.2262) centre (-19.3034, -30.7262) ccw
  line L75 (-18.8034, -34.1903) -> (-18.8034, -34.7262)
  line L76 (-19.8034, -34.7262) -> (-18.8034, -34.7262)
  line L77 (-19.8034, -34.7262) -> (-19.8034, -34.1903)
  arc A41 (-22.7675, -31.2262) -> (-19.8034, -34.1903) centre (-19.3034, -30.7262) ccw
  line L78 (-22.7675, -31.2262) -> (-23.8034, -31.2262)
  line L79 (-23.8034, -30.2262) -> (-23.8034, -31.2262)
  line L80 (-23.8034, -30.2262) -> (-22.7675, -30.2262)
  arc A42 (-19.8034, -27.2621) -> (-22.7675, -30.2262) centre (-19.3034, -30.7262) ccw
  line L81 (-19.8034, -27.2621) -> (-19.8034, -24.1903)
  arc A43 (-22.7675, -21.2262) -> (-19.8034, -24.1903) centre (-19.3034, -20.7262) ccw
  line L82 (-22.7675, -21.2262) -> (-23.8034, -21.2262)
  line L83 (-23.8034, -20.2262) -> (-23.8034, -21.2262)
  line L84 (-23.8034, -20.2262) -> (-22.7675, -20.2262)
  arc A44 (-19.8034, -17.2621) -> (-22.7675, -20.2262) centre (-19.3034, -20.7262) ccw
  line L85 (-19.8034, -17.2621) -> (-19.8034, -14.1903)
  arc A45 (-22.7675, -11.2262) -> (-19.8034, -14.1903) centre (-19.3034, -10.7262) ccw
  line L86 (-22.7675, -11.2262) -> (-23.8034, -11.2262)
  line L87 (-23.8034, -10.2262) -> (-23.8034, -11.2262)
  line L88 (-23.8034, -10.2262) -> (-22.7675, -10.2262)
  arc A46 (-19.8034, -7.2621) -> (-22.7675, -10.2262) centre (-19.3034, -10.7262) ccw
  line L89 (-19.8034, -7.2621) -> (-19.8034, -4.1903)
  arc A47 (-22.7675, -1.2262) -> (-19.8034, -4.1903) centre (-19.3034, -0.7262) ccw
  line L90 (-22.7675, -1.2262) -> (-23.8034, -1.2262)
  line L91 (-23.8034, -0.2262) -> (-23.8034, -1.2262)
  circle A48 centre (-19.3034, -10.7262) radius 2.5
  circle A49 centre (-19.3034, -20.7262) radius 2.5
  circle A50 centre (-19.3034, -30.7262) radius 2.5
  circle A51 centre (-19.3034, -0.7262) radius 2.5
  line L92 (-13.8034, -0.2262) -> (-12.7675, -0.2262)
  arc A52 (-9.8034, 2.7379) -> (-12.7675, -0.2262) centre (-9.3034, -0.7262) ccw
  line L93 (-9.8034, 2.7379) -> (-9.8034, 3.2738)
  line L94 (-8.8034, 3.2738) -> (-9.8034, 3.2738)
  line L95 (-8.8034, 3.2738) -> (-8.8034, 2.7379)
  arc A53 (-5.8393, -0.2262) -> (-8.8034, 2.7379) centre (-9.3034, -0.7262) ccw
  line L96 (-5.8393, -0.2262) -> (-4.8034, -0.2262)
  line L97 (-4.8034, -1.2262) -> (-4.8034, -0.2262)
  line L98 (-4.8034, -1.2262) -> (-5.8393, -1.2262)
  arc A54 (-8.8034, -4.1903) -> (-5.8393, -1.2262) centre (-9.3034, -0.7262) ccw
  line L99 (-8.8034, -4.1903) -> (-8.8034, -7.2621)
  arc A55 (-5.8393, -10.2262) -> (-8.8034, -7.2621) centre (-9.3034, -10.7262) ccw
  line L100 (-5.8393, -10.2262) -> (-4.8034, -10.2262)
  line L101 (-4.8034, -11.2262) -> (-4.8034, -10.2262)
  line L102 (-4.8034, -11.2262) -> (-5.8393, -11.2262)
  arc A56 (-8.8034, -14.1903) -> (-5.8393, -11.2262) centre (-9.3034, -10.7262) ccw
  line L103 (-8.8034, -14.1903) -> (-8.8034, -17.2621)
  arc A57 (-5.8393, -20.2262) -> (-8.8034, -17.2621) centre (-9.3034, -20.7262) ccw
  line L104 (-5.8393, -20.2262) -> (-4.8034, -20.2262)
  line L105 (-4.8034, -21.2262) -> (-4.8034, -20.2262)
  line L106 (-4.8034, -21.2262) -> (-5.8393, -21.2262)
  arc A58 (-8.8034, -24.1903) -> (-5.8393, -21.2262) centre (-9.3034, -20.7262) ccw
  line L107 (-8.8034, -24.1903) -> (-8.8034, -27.2621)
  arc A59 (-5.8393, -30.2262) -> (-8.8034, -27.2621) centre (-9.3034, -30.7262) ccw
  line L108 (-5.8393, -30.2262) -> (-4.8034, -30.2262)
  line L109 (-4.8034, -31.2262) -> (-4.8034, -30.2262)
  line L110 (-4.8034, -31.2262) -> (-5.8393, -31.2262)
  arc A60 (-8.8034, -34.1903) -> (-5.8393, -31.2262) centre (-9.3034, -30.7262) ccw
  line L111 (-8.8034, -34.1903) -> (-8.8034, -34.7262)
  line L112 (-9.8034, -34.7262) -> (-8.8034, -34.7262)
  line L113 (-9.8034, -34.7262) -> (-9.8034, -34.1903)
  arc A61 (-12.7675, -31.2262) -> (-9.8034, -34.1903) centre (-9.3034, -30.7262) ccw
  line L114 (-12.7675, -31.2262) -> (-13.8034, -31.2262)
  line L115 (-13.8034, -30.2262) -> (-13.8034, -31.2262)
  line L116 (-13.8034, -30.2262) -> (-12.7675, -30.2262)
  arc A62 (-9.8034, -27.2621) -> (-12.7675, -30.2262) centre (-9.3034, -30.7262) ccw
  line L117 (-9.8034, -27.2621) -> (-9.8034, -24.1903)
  arc A63 (-12.7675, -21.2262) -> (-9.8034, -24.1903) centre (-9.3034, -20.7262) ccw
  line L118 (-12.7675, -21.2262) -> (-13.8034, -21.2262)
  line L119 (-13.8034, -20.2262) -> (-13.8034, -21.2262)
  line L120 (-13.8034, -20.2262) -> (-12.7675, -20.2262)
  arc A64 (-9.8034, -17.2621) -> (-12.7675, -20.2262) centre (-9.3034, -20.7262) ccw
  line L121 (-9.8034, -17.2621) -> (-9.8034, -14.1903)
  arc A65 (-12.7675, -11.2262) -> (-9.8034, -14.1903) centre (-9.3034, -10.7262) ccw
  line L122 (-12.7675, -11.2262) -> (-13.8034, -11.2262)
  line L123 (-13.8034, -10.2262) -> (-13.8034, -11.2262)
  line L124 (-13.8034, -10.2262) -> (-12.7675, -10.2262)
  arc A66 (-9.8034, -7.2621) -> (-12.7675, -10.2262) centre (-9.3034, -10.7262) ccw
  line L125 (-9.8034, -7.2621) -> (-9.8034, -4.1903)
  arc A67 (-12.7675, -1.2262) -> (-9.8034, -4.1903) centre (-9.3034, -0.7262) ccw
  line L126 (-12.7675, -1.2262) -> (-13.8034, -1.2262)
  line L127 (-13.8034, -0.2262) -> (-13.8034, -1.2262)
  circle A68 centre (-9.3034, -10.7262) radius 2.5
  circle A69 centre (-9.3034, -20.7262) radius 2.5
  circle A70 centre (-9.3034, -30.7262) radius 2.5
  circle A71 centre (-9.3034, -0.7262) radius 2.5
  line L128 (0.1966, -7.2621) -> (0.1966, -4.1903)
  arc A72 (-2.7675, -1.2262) -> (0.1966, -4.1903) centre (0.6966, -0.7262) ccw
  line L129 (-2.7675, -1.2262) -> (-3.8034, -1.2262)
  line L130 (-3.8034, -0.2262) -> (-3.8034, -1.2262)
  line L131 (-3.8034, -0.2262) -> (-2.7675, -0.2262)
  arc A73 (0.1966, 2.7379) -> (-2.7675, -0.2262) centre (0.6966, -0.7262) ccw
  line L132 (0.1966, 2.7379) -> (0.1966, 3.2738)
  line L133 (0.6966, 3.2738) -> (0.1966, 3.2738)
  arc A74 (1.1966, 3.2424) -> (0.6966, 3.2738) centre (0.6966, -0.7262) ccw
  line L134 (1.1966, 3.2424) -> (1.1966, 2.7379)
  arc A75 (4.1607, -0.2262) -> (1.1966, 2.7379) centre (0.6966, -0.7262) ccw
  line L135 (4.1607, -0.2262) -> (4.6652, -0.2262)
  arc A76 (4.6966, -0.7262) -> (4.6652, -0.2262) centre (0.6966, -0.7262) ccw
  line L136 (4.6966, -1.2262) -> (4.6966, -0.7262)
  line L137 (4.6966, -1.2262) -> (4.1607, -1.2262)
  arc A77 (1.1966, -4.1903) -> (4.1607, -1.2262) centre (0.6966, -0.7262) ccw
  line L138 (1.1966, -4.1903) -> (1.1966, -7.2621)
  arc A78 (4.1607, -10.2262) -> (1.1966, -7.2621) centre (0.6966, -10.7262) ccw
  line L139 (4.1607, -10.2262) -> (4.6966, -10.2262)
  line L140 (4.6966, -11.2262) -> (4.6966, -10.2262)
  line L141 (4.6966, -11.2262) -> (4.1607, -11.2262)
  arc A79 (1.1966, -14.1903) -> (4.1607, -11.2262) centre (0.6966, -10.7262) ccw
  line L142 (1.1966, -14.1903) -> (1.1966, -17.2621)
  arc A80 (4.1607, -20.2262) -> (1.1966, -17.2621) centre (0.6966, -20.7262) ccw
  line L143 (4.1607, -20.2262) -> (4.6966, -20.2262)
  line L144 (4.6966, -21.2262) -> (4.6966, -20.2262)
  line L145 (4.6966, -21.2262) -> (4.1607, -21.2262)
  arc A81 (1.1966, -24.1903) -> (4.1607, -21.2262) centre (0.6966, -20.7262) ccw
  line L146 (1.1966, -24.1903) -> (1.1966, -27.2621)
  arc A82 (4.1607, -30.2262) -> (1.1966, -27.2621) centre (0.6966, -30.7262) ccw
  line L147 (4.1607, -30.2262) -> (4.6966, -30.2262)
  line L148 (4.6966, -30.7262) -> (4.6966, -30.2262)
  arc A83 (4.6652, -31.2262) -> (4.6966, -30.7262) centre (0.6966, -30.7262) ccw
  line L149 (4.6652, -31.2262) -> (4.1607, -31.2262)
  arc A84 (1.1966, -34.1903) -> (4.1607, -31.2262) centre (0.6966, -30.7262) ccw
  line L150 (1.1966, -34.1903) -> (1.1966, -34.6949)
  arc A85 (0.6966, -34.7262) -> (1.1966, -34.6949) centre (0.6966, -30.7262) ccw
  line L151 (0.1966, -34.7262) -> (0.6966, -34.7262)
  line L152 (0.1966, -34.7262) -> (0.1966, -34.1903)
  arc A86 (-2.7675, -31.2262) -> (0.1966, -34.1903) centre (0.6966, -30.7262) ccw
  line L153 (-2.7675, -31.2262) -> (-3.8034, -31.2262)
  line L154 (-3.8034, -30.2262) -> (-3.8034, -31.2262)
  line L155 (-3.8034, -30.2262) -> (-2.7675, -30.2262)
  arc A87 (0.1966, -27.2621) -> (-2.7675, -30.2262) centre (0.6966, -30.7262) ccw
  line L156 (0.1966, -27.2621) -> (0.1966, -24.1903)
  arc A88 (-2.7675, -21.2262) -> (0.1966, -24.1903) centre (0.6966, -20.7262) ccw
  line L157 (-2.7675, -21.2262) -> (-3.8034, -21.2262)
  line L158 (-3.8034, -20.2262) -> (-3.8034, -21.2262)
  line L159 (-3.8034, -20.2262) -> (-2.7675, -20.2262)
  arc A89 (0.1966, -17.2621) -> (-2.7675, -20.2262) centre (0.6966, -20.7262) ccw
  line L160 (0.1966, -17.2621) -> (0.1966, -14.1903)
  arc A90 (-2.7675, -11.2262) -> (0.1966, -14.1903) centre (0.6966, -10.7262) ccw
  line L161 (-2.7675, -11.2262) -> (-3.8034, -11.2262)
  line L162 (-3.8034, -10.2262) -> (-3.8034, -11.2262)
  line L163 (-3.8034, -10.2262) -> (-2.7675, -10.2262)
  arc A91 (0.1966, -7.2621) -> (-2.7675, -10.2262) centre (0.6966, -10.7262) ccw
  circle A92 centre (0.6966, -10.7262) radius 2.5
  circle A93 centre (0.6966, -20.7262) radius 2.5
  circle A94 centre (0.6966, -30.7262) radius 2.5
  circle A95 centre (0.6966, -0.7262) radius 2.5
  point P0 (90.2539, -56.452)
  constraints: 316 end point, 160 point on circle, 96 centre point, 18 other
extrude "Extrusion6" cut sketch "Sketch3" against normal blind 6.8 contours A5 L149 A84 L150 L7 L152 A86 L153 L6 L155 A87 L156 A88 L157 L159 A89 L160 A90 L161 L163 A91 L128 A72 L129 L131 A73 L132 L5 A4 L134 A75 L135 L4 L137 A77 L138 A78 L139 L141 A79 L142 A80 L143 L145 A81 L146 A82 L147 | L147 A82 L146 A81 L145 L4 | A5 L150 A84 L149 | L143 A80 L142 A79 L141 L4 | L7 L6 L153 A86 L152 | L139 A78 L138 A77 L137 L4 | L6 L157 A88 L156 A87 L155 | L135 A75 L134 A4 | L6 L161 A90 L160 A89 L159 | L132 A73 L131 L6 L5 | L6 L129 A72 L128 A91 L163 | L11 L114 A61 L113 L8 | L113 A61 L114 L11 L116 A62 L117 A63 L118 L120 A64 L121 A65 L122 L124 A66 L125 A67 L126 L92 A52 L93 L10 L95 A53 L96 L9 L98 A54 L99 A55 L100 L102 A56 L103 A57 L104 L106 A58 L107 A59 L108 L110 A60 L111 L8 | L111 A60 L110 L9 L8 | L11 L118 A63 L117 A62 L116 | L11 L122 A65 L121 A64 L120 | L108 A59 L107 A58 L106 L9 | L11 L126 A67 L125 A66 L124 | L104 A57 L103 A56 L102 L9 | L11 L10 L93 A52 L92 | L100 A55 L99 A54 L98 L9 | L96 A53 L95 L10 L9 | L15 L78 A41 L77 L12 | L77 A41 L78 L15 L80 A42 L81 A43 L82 L84 A44 L85 A45 L86 L88 A46 L89 A47 L90 L56 A32 L57 L14 L59 A33 L60 L13 L62 A34 L63 A35 L64 L66 A36 L67 A37 L68 L70 A38 L71 A39 L72 L74 A40 L75 L12 | L75 A40 L74 L13 L12 | L15 L82 A43 L81 A42 L80 | L15 L86 A45 L85 A44 L84 | L72 A39 L71 A38 L70 L13 | L15 L90 A47 L89 A46 L88 | L68 A37 L67 A36 L66 L13 | L15 L14 L57 A32 L56 | L64 A35 L63 A34 L62 L13 | L60 A33 L59 L14 L13 | A7 L49 A24 L50 L19 L52 A26 L53 L18 L55 A27 L20 A8 L21 L23 A9 L24 A10 L25 L27 A11 L28 A12 L29 L31 A13 L32 L17 A6 L34 A15 L35 L16 L37 A17 L38 A18 L39 L41 A19 L42 A20 L43 L45 A21 L46 A22 L47 | L47 A22 L46 A21 L45 L16 | A7 L50 A24 L49 | L43 A20 L42 A19 L41 L16 | L19 L18 L53 A26 L52 | L39 A18 L38 A17 L37 L16 | L18 L21 A8 L20 A27 L55 | L35 A15 L34 A6 | L18 L25 A10 L24 A9 L23 | L32 A13 L31 L18 L17 | L18 L29 A12 L28 A11 L27 | A28 | A29 | A30 | A31 | A48 | A49 | A50 | A51 | A68 | A69 | A70 | A71 | A92 | A93 | A94 | A95
sketch "Sketch4" plane through (-90.2539, 56.452, 16) normal (0, 0, 1) x (1, 0, 0)
  line L0 (-4.8034, -34.7262) -> (-13.8034, -34.7262) projected
  line L1 (-13.8034, -34.7262) -> (-13.8034, 3.2738) projected
  line L2 (-13.8034, 3.2738) -> (-4.8034, 3.2738) projected
  line L3 (-4.8034, 3.2738) -> (-4.8034, -34.7262) projected
  line L4 (4.6966, -0.7262) -> (4.6966, -30.7262) projected
  arc A0 (0.6966, -34.7262) -> (4.6966, -30.7262) centre (0.6966, -30.7262) ccw projected
  line L5 (0.6966, -34.7262) -> (-3.8034, -34.7262) projected
  line L6 (-3.8034, -34.7262) -> (-3.8034, 3.2738) projected
  line L7 (-3.8034, 3.2738) -> (0.6966, 3.2738) projected
  arc A1 (4.6966, -0.7262) -> (0.6966, 3.2738) centre (0.6966, -0.7262) ccw projected
  line L8 (-33.3034, -30.7262) -> (-33.3034, -0.7262) projected
  arc A2 (-29.3034, 3.2738) -> (-33.3034, -0.7262) centre (-29.3034, -0.7262) ccw projected
  line L9 (-29.3034, 3.2738) -> (-24.8034, 3.2738) projected
  line L10 (-24.8034, 3.2738) -> (-24.8034, -34.7262) projected
  line L11 (-24.8034, -34.7262) -> (-29.3034, -34.7262) projected
  arc A3 (-33.3034, -30.7262) -> (-29.3034, -34.7262) centre (-29.3034, -30.7262) ccw projected
  line L12 (-14.8034, -34.7262) -> (-23.8034, -34.7262) projected
  line L13 (-23.8034, -34.7262) -> (-23.8034, 3.2738) projected
  line L14 (-23.8034, 3.2738) -> (-14.8034, 3.2738) projected
  line L15 (-14.8034, 3.2738) -> (-14.8034, -34.7262) projected
  arc A4 (0.6966, -35.7262) -> (5.6966, -30.7262) centre (0.6966, -30.7262) ccw projected
  line L16 (5.6966, -30.7262) -> (5.6966, -0.7262) projected
  arc A5 (5.6966, -0.7262) -> (0.6966, 4.2738) centre (0.6966, -0.7262) ccw projected
  line L17 (0.6966, 4.2738) -> (-29.3034, 4.2738) projected
  arc A6 (-29.3034, 4.2738) -> (-34.3034, -0.7262) centre (-29.3034, -0.7262) ccw projected
  line L18 (-34.3034, -0.7262) -> (-34.3034, -30.7262) projected
  arc A7 (-34.3034, -30.7262) -> (-29.3034, -35.7262) centre (-29.3034, -30.7262) ccw projected
  line L19 (-29.3034, -35.7262) -> (0.6966, -35.7262) projected
  circle A8 centre (-14.3034, -15.7262) radius 15.5
  circle A9 centre (-27.9152, -29.338) radius 2
  circle A10 centre (-0.6916, -2.1144) radius 2
  arc A11 (3.9968, -2.877) -> (-1.4542, 2.574) centre (-0.6916, -2.1144) ccw
  line L20 (-1.4542, 2.574) -> (-16.8721, 0.0662)
  arc A12 (-16.8721, 0.0662) -> (-30.0959, -13.1576) centre (-14.3034, -15.7262) ccw
  line L21 (-30.0959, -13.1576) -> (-32.6036, -28.5755)
  arc A13 (-32.6036, -28.5755) -> (-27.1526, -34.0264) centre (-27.9152, -29.338) ccw
  line L22 (-27.1526, -34.0264) -> (-11.7347, -31.5187)
  arc A14 (-11.7347, -31.5187) -> (1.4891, -18.2949) centre (-14.3034, -15.7262) ccw
  line L23 (1.4891, -18.2949) -> (3.9968, -2.877)
  line L24 (-3.8034, -6.7262) -> (4.6966, -6.7262)
  line L25 (-33.3034, -24.7262) -> (-24.8034, -24.7262)
  line L26 (-24.8034, -34.7262) -> (-29.3034, -34.7262) projected
  line L27 (-3.8034, 3.2738) -> (0.6966, 3.2738) projected
  point P0 (90.2539, -56.452)
  dimension "d12" = 10
  dimension "d13" = 10
  constraints: 12 end point, 8 point on circle, 7 centre point, 4 point on line, 2 parallel
  measures "d12" distance between parallel lines of L24 L7
  measures "d13" distance between parallel lines of L11 L25
ref_plane "Work Plane2" through (-124.5573, 20.7257, 0) normal (0, 0, 1) x (1, 0, 0)
extrude "Extrusion7" add sketch "Sketch4" against normal up to surface (16 mm away) contours A8 L24 L6 | L6 L20 A11 L23 L24 A8 | L23 A11 L20 L6 L7 A1 L4 L24 | L22 A13 L21 L25 A8 L10 | L10 L11 A3 L8 L25 L21 A13 L22 | A8 L25 L10 picked at (-3.5497, -5.3754) picked at (-25.0571, -26.077)
sketch "Sketch5" plane through (-90.2539, 56.452, 16) normal (0, 0, 1) x (1, 0, 0)
  circle A0 centre (-27.9152, -29.338) radius 2 projected
  circle A1 centre (-0.6916, -2.1144) radius 2 projected
  line L0 (-4.8034, -34.7262) -> (-13.8034, -34.7262) projected
  line L1 (-13.8034, -34.7262) -> (-13.8034, 3.2738) projected
  line L2 (-13.8034, 3.2738) -> (-4.8034, 3.2738) projected
  line L3 (-4.8034, 3.2738) -> (-4.8034, -34.7262) projected
  line L4 (4.6966, -6.7262) -> (4.6966, -30.7262) projected
  arc A2 (0.6966, -34.7262) -> (4.6966, -30.7262) centre (0.6966, -30.7262) ccw projected
  line L5 (0.6966, -34.7262) -> (-3.8034, -34.7262) projected
  line L6 (-3.8034, -34.7262) -> (-3.8034, -6.7262) projected
  line L7 (-3.8034, -6.7262) -> (4.6966, -6.7262) projected
  line L8 (-33.3034, -24.7262) -> (-33.3034, -0.7262) projected
  arc A3 (-29.3034, 3.2738) -> (-33.3034, -0.7262) centre (-29.3034, -0.7262) ccw projected
  line L9 (-29.3034, 3.2738) -> (-24.8034, 3.2738) projected
  line L10 (-24.8034, 3.2738) -> (-24.8034, -24.7262) projected
  line L11 (-24.8034, -24.7262) -> (-33.3034, -24.7262) projected
  line L12 (-14.8034, -34.7262) -> (-23.8034, -34.7262) projected
  line L13 (-23.8034, -34.7262) -> (-23.8034, 3.2738) projected
  line L14 (-23.8034, 3.2738) -> (-14.8034, 3.2738) projected
  line L15 (-14.8034, 3.2738) -> (-14.8034, -34.7262) projected
  arc A4 (0.6966, -35.7262) -> (5.6966, -30.7262) centre (0.6966, -30.7262) ccw projected
  line L16 (5.6966, -30.7262) -> (5.6966, -0.7262) projected
  arc A5 (5.6966, -0.7262) -> (0.6966, 4.2738) centre (0.6966, -0.7262) ccw projected
  line L17 (0.6966, 4.2738) -> (-29.3034, 4.2738) projected
  arc A6 (-29.3034, 4.2738) -> (-34.3034, -0.7262) centre (-29.3034, -0.7262) ccw projected
  line L18 (-34.3034, -0.7262) -> (-34.3034, -30.7262) projected
  arc A7 (-34.3034, -30.7262) -> (-29.3034, -35.7262) centre (-29.3034, -30.7262) ccw projected
  line L19 (-29.3034, -35.7262) -> (0.6966, -35.7262) projected
  point P0 (90.2539, -56.452)
extrude "Extrusion8" cut sketch "Sketch5" against normal through all contours A0 | A1
sketch "Sketch6" plane through (-90.2539, 56.452, 0) normal (0, 0, -1) x (-1, 0, 0)
  circle A0 centre (27.9152, -29.338) radius 2
  circle A1 centre (0.6916, -2.1144) radius 2
  line L0 (13.8034, -34.7262) -> (4.8034, -34.7262)
  line L1 (4.8034, -34.7262) -> (4.8034, 3.2738)
  line L2 (4.8034, 3.2738) -> (13.8034, 3.2738)
  line L3 (13.8034, 3.2738) -> (13.8034, -34.7262)
  line L4 (-4.6966, -30.7262) -> (-4.6966, -6.7262)
  line L5 (-4.6966, -6.7262) -> (3.8034, -6.7262)
  line L6 (3.8034, -6.7262) -> (3.8034, -34.7262)
  line L7 (3.8034, -34.7262) -> (-0.6966, -34.7262)
  arc A2 (-4.6966, -30.7262) -> (-0.6966, -34.7262) centre (-0.6966, -30.7262) ccw
  line L8 (33.3034, -0.7262) -> (33.3034, -24.7262)
  line L9 (33.3034, -24.7262) -> (24.8034, -24.7262)
  line L10 (24.8034, -24.7262) -> (24.8034, 3.2738)
  line L11 (24.8034, 3.2738) -> (29.3034, 3.2738)
  arc A3 (33.3034, -0.7262) -> (29.3034, 3.2738) centre (29.3034, -0.7262) ccw
  line L12 (23.8034, -34.7262) -> (14.8034, -34.7262)
  line L13 (14.8034, -34.7262) -> (14.8034, 3.2738)
  line L14 (14.8034, 3.2738) -> (23.8034, 3.2738)
  line L15 (23.8034, 3.2738) -> (23.8034, -34.7262)
  arc A4 (-5.6966, -30.7262) -> (-0.6966, -35.7262) centre (-0.6966, -30.7262) ccw
  line L16 (29.3034, -35.7262) -> (-0.6966, -35.7262)
  arc A5 (29.3034, -35.7262) -> (34.3034, -30.7262) centre (29.3034, -30.7262) ccw
  line L17 (34.3034, -0.7262) -> (34.3034, -30.7262)
  arc A6 (34.3034, -0.7262) -> (29.3034, 4.2738) centre (29.3034, -0.7262) ccw
  line L18 (-0.6966, 4.2738) -> (29.3034, 4.2738)
  arc A7 (-0.6966, 4.2738) -> (-5.6966, -0.7262) centre (-0.6966, -0.7262) ccw
  line L19 (-5.6966, -30.7262) -> (-5.6966, -0.7262)
  line L20 (3.8034, -6.7262) -> (-4.6966, -6.7262)
  line L21 (3.8034, -6.7262) -> (4.8034, -6.7262)
  line L22 (24.8034, -24.7262) -> (23.8034, -24.7262)
  line L23 (24.8034, -24.7262) -> (33.3034, -24.7262)
  line L24 (33.3034, -24.7262) -> (34.3034, -24.7262)
  line L25 (23.8034, -34.7262) -> (23.8034, -35.7262)
  line L26 (-4.6966, -6.7262) -> (-5.6966, -6.7262)
  line L27 (4.8034, 3.2738) -> (4.8034, 4.2738)
  line L28 (33.3034, -0.7262) -> (33.3034, -30.7262)
  arc A8 (29.3034, -34.7262) -> (33.3034, -30.7262) centre (29.3034, -30.7262) ccw
  line L29 (29.3034, -34.7262) -> (24.8034, -34.7262)
  line L30 (-4.6966, -30.7262) -> (-4.6966, -0.7262)
  arc A9 (-0.6966, 3.2738) -> (-4.6966, -0.7262) centre (-0.6966, -0.7262) ccw
  line L31 (-0.6966, 3.2738) -> (3.8034, 3.2738)
  line L32 (24.8034, -34.7262) -> (23.8034, -34.7262)
  line L33 (4.8034, 3.2738) -> (3.8034, 3.2738)
  point P0 (-90.2539, -56.452)
extrude "Extrusion9" cut sketch "Sketch6" against normal blind 5 contours L21 L5 L30 A9 L31 L33 L1 | L28 A8 L29 L32 L15 L22 L9
equation "\"d13\" = d12"
body "Solid2"
